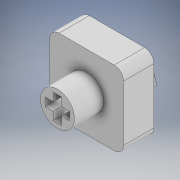
# Autodesk Inventor part: IPC ALOW 2 key
Saved by Autodesk Inventor 2022 (Build 260153000, 153)
## iProperties
Created: 2021-12-31
Part Number: IPC ALOW 2 key
Material: Generic
Document SubType Name: Modeling
Designer: solor
Density: 1 g/cm^3
Appearance: Default
Author: solor
Autodesk Inventor part; units mm, degrees
ref_plane "YZ Plane" through (0, 0, 0) normal (1, 0, 0) x (0, 1, 0)
ref_plane "XZ Plane" through (0, 0, 0) normal (0, 1, 0) x (-1, 0, 0)
sketch "Sketch1" plane through (0, 0, 0) normal (0, 0, 1) x (1, 0, 0)
  line L0 (14.6962, 12.74) -> (14.6962, 0) construction
  line L1 (10.61, 12.2) -> (1.53, 12.2)
  arc A0 (1.53, 12.2) -> (0, 10.67) centre (1.53, 10.67) ccw
  line L2 (0, 10.67) -> (0, 1.53)
  arc A1 (0, 1.53) -> (1.53, 0) centre (1.53, 1.53) ccw
  line L3 (1.53, 0) -> (10.61, 0)
  arc A2 (10.61, 0) -> (12.14, 1.53) centre (10.61, 1.53) ccw
  arc A3 (12.14, 10.67) -> (10.61, 12.2) centre (10.61, 10.67) ccw
  line L4 (12.14, 10.67) -> (12.14, 1.53)
  point P0 (0, 0)
  point P1 (0, 0)
  dimension "d10" = 12.74
  constraints: 10 end point, 8 point on circle, 4 centre point, 2 vertical, 1 point on line
  measures "d10" distance of L0.start L0.end
ref_plane "Work Plane1" through (0, 0, 5) normal (0, 0, 1) x (1, 0, 0)
sketch "Sketch2" plane through (0, 0, 5) normal (0, 0, 1) x (1, 0, 0)
  line L0 (10.88, 12.74) -> (1.8, 12.74) projected
  line L1 (10.88, 12.74) -> (1.8, 12.74) projected
  arc A0 (1.8, 12.74) -> (0, 10.94) centre (1.8, 10.94) ccw projected
  line L2 (0, 10.94) -> (0, 1.8) projected
  arc A1 (0, 1.8) -> (1.8, 0) centre (1.8, 1.8) ccw projected
  line L3 (1.8, 0) -> (10.88, 0) projected
  arc A2 (10.88, 0) -> (12.68, 1.8) centre (10.88, 1.8) ccw projected
  line L4 (12.68, 1.8) -> (12.68, 10.94) projected
  arc A3 (12.68, 10.94) -> (10.88, 12.74) centre (10.88, 10.94) ccw projected
  circle A4 centre (6.34, 6.37) radius 2.8
  line L5 (5.665, 8.395) -> (7.015, 8.395)
  line L6 (7.015, 4.345) -> (5.665, 4.345)
  line L7 (5.665, 4.345) -> (7.015, 8.395) construction
  line L8 (5.665, 8.395) -> (7.015, 4.345) construction
  line L9 (8.365, 5.695) -> (8.365, 7.045)
  line L10 (4.315, 7.045) -> (4.315, 5.695)
  line L11 (4.315, 5.695) -> (8.365, 7.045) construction
  line L12 (8.365, 5.695) -> (4.315, 7.045) construction
  line L13 (4.315, 5.695) -> (5.665, 5.695)
  line L14 (7.015, 5.695) -> (8.365, 5.695)
  line L15 (5.665, 4.345) -> (5.665, 5.695)
  line L16 (5.665, 7.045) -> (5.665, 8.395)
  line L17 (8.365, 7.045) -> (7.015, 7.045)
  line L18 (5.665, 7.045) -> (4.315, 7.045)
  line L19 (7.015, 8.395) -> (7.015, 7.045)
  line L20 (7.015, 5.695) -> (7.015, 4.345)
  point P0 (0, 0)
  dimension "d3" = 5.6
  dimension "d4" = 4.05
  dimension "d5" = 1.35
  dimension "d6" = 4.05
  dimension "d7" = 1.35
  constraints: 32 end point, 10 parallel, 8 perpendicular, 4 midpoint, 2 vertical, 1 centre point
  measures "d3" diameter of A4
  measures "d4" distance of L6.end L5.start
  measures "d5" distance of L5.start L5.end
  measures "d6" distance of L10.end L9.start
  measures "d7" distance of L9.end L9.start
extrude "Extrusion3" add sketch "Sketch1" along normal blind 5
sketch "Sketch3" plane through (0, 0, 5) normal (0, 0, 1) x (1, 0, 0)
  line L0 (10.61, 12.47) -> (1.53, 12.47)
  line L1 (10.61, 12.47) -> (1.53, 12.47)
  arc A0 (1.53, 12.47) -> (-0.27, 10.67) centre (1.53, 10.67) ccw
  line L2 (-0.27, 10.67) -> (-0.27, 1.53)
  arc A1 (-0.27, 1.53) -> (1.53, -0.27) centre (1.53, 1.53) ccw
  line L3 (1.53, -0.27) -> (10.61, -0.27)
  arc A2 (10.61, -0.27) -> (12.41, 1.53) centre (10.61, 1.53) ccw
  line L4 (12.41, 1.53) -> (12.41, 10.67)
  arc A3 (12.41, 10.67) -> (10.61, 12.47) centre (10.61, 10.67) ccw
  circle A4 centre (6.07, 6.1) radius 2.8
  line L5 (5.395, 8.125) -> (6.745, 8.125)
  line L6 (6.745, 4.075) -> (5.395, 4.075)
  line L7 (5.395, 4.075) -> (6.745, 8.125) construction
  line L8 (5.395, 8.125) -> (6.745, 4.075) construction
  line L9 (8.095, 5.425) -> (8.095, 6.775)
  line L10 (4.045, 6.775) -> (4.045, 5.425)
  line L11 (4.045, 5.425) -> (8.095, 6.775) construction
  line L12 (8.095, 5.425) -> (4.045, 6.775) construction
  line L13 (4.045, 5.425) -> (5.395, 5.425)
  line L14 (6.745, 5.425) -> (8.095, 5.425)
  line L15 (5.395, 4.075) -> (5.395, 5.425)
  line L16 (5.395, 6.775) -> (5.395, 8.125)
  line L17 (8.095, 6.775) -> (6.745, 6.775)
  line L18 (5.395, 6.775) -> (4.045, 6.775)
  line L19 (6.745, 8.125) -> (6.745, 6.775)
  line L20 (6.745, 5.425) -> (6.745, 4.075)
  line L21 (10.61, 12.2) -> (1.53, 12.2) projected
  line L22 (0, 10.67) -> (0, 1.53) projected
  point P0 (0, 0)
  point P1 (-0.27, -0.27)
  point P2 (6.07, 12.2)
  point P3 (0, 6.1)
  point P4 (6.07, 6.1)
  dimension "d14" = 5.6
  dimension "d15" = 4.05
  dimension "d16" = 1.35
  dimension "d17" = 4.05
  dimension "d18" = 1.35
  constraints: 42 end point, 10 parallel, 8 perpendicular, 8 point on circle, 6 midpoint, 5 centre point, 2 vertical
  measures "d14" diameter of A4
  measures "d15" distance of L6.end L5.start
  measures "d16" distance of L5.start L5.end
  measures "d17" distance of L10.end L9.start
  measures "d18" distance of L9.end L9.start
extrude "Extrusion4" add sketch "Sketch3" along normal blind 4.8 contours A4
sketch "Sketch4" plane through (0, 0, 0) normal (0, 0, -1) x (-1, 0, 0)
  line L0 (-1.53, 0) -> (-10.61, 0) projected
  line L1 (-11.7223, 9.7129) -> (-0.4177, 9.7129) construction
  line L2 (-0.4177, 9.7129) -> (-0.4177, 6.84) construction
  line L3 (-0.4177, 6.84) -> (-11.7223, 6.84) construction
  line L4 (-11.7223, 6.84) -> (-11.7223, 9.7129) construction
  line L5 (-7.4059, 5.3753) -> (-4.7341, 5.3753) construction
  line L6 (-4.7341, 5.3753) -> (-4.7341, 2.266) construction
  line L7 (-4.7341, 2.266) -> (-7.4059, 2.266) construction
  line L8 (-7.4059, 2.266) -> (-7.4059, 5.3753) construction
  line L9 (-11.7333, 6.956) -> (-10.8209, 9.656)
  line L10 (-10.8209, 9.656) -> (-10.0813, 9.656)
  line L11 (-10.0813, 9.656) -> (-9.1689, 6.956)
  line L12 (-9.1689, 6.956) -> (-9.8669, 6.956)
  line L13 (-9.8669, 6.956) -> (-10.0354, 7.5074)
  line L14 (-10.0354, 7.5074) -> (-10.8843, 7.5074)
  line L15 (-10.8843, 7.5074) -> (-11.055, 6.956)
  line L16 (-11.055, 6.956) -> (-11.7333, 6.956)
  line L17 (-10.1842, 7.9975) -> (-10.4598, 8.8902)
  line L18 (-10.4598, 8.8902) -> (-10.7377, 7.9975)
  line L19 (-10.7377, 7.9975) -> (-10.1842, 7.9975)
  line L20 (-7.0991, 6.956) -> (-8.8998, 6.956)
  line L21 (-8.8998, 6.956) -> (-8.8998, 9.656)
  line L22 (-8.8998, 9.656) -> (-8.2215, 9.656)
  line L23 (-8.2215, 9.656) -> (-8.2215, 7.4702)
  line L24 (-8.2215, 7.4702) -> (-7.0991, 7.4702)
  line L25 (-7.0991, 7.4702) -> (-7.0991, 6.956)
  spline S0 degree 2 poles (-4.3181, 8.306) (-4.3181, 7.6496) (-5.0183, 6.8991) (-5.6265, 6.8991) knots 0 0 0 1 2 2 2
  spline S1 degree 2 poles (-5.6265, 6.8991) (-6.237, 6.8991) (-6.9328, 7.6584) (-6.9328, 8.306) knots 0 0 0 1 2 2 2
  spline S2 degree 2 poles (-6.9328, 8.306) (-6.9328, 8.9559) (-6.237, 9.7129) (-5.6265, 9.7129) knots 0 0 0 1 2 2 2
  spline S3 degree 2 poles (-5.6265, 9.7129) (-5.0183, 9.7129) (-4.3181, 8.9602) (-4.3181, 8.306) knots 0 0 0 1 2 2 2
  spline S4 degree 2 poles (-5.0183, 8.306) (-5.0183, 8.5489) (-5.1167, 8.888) (-5.2021, 8.9952) knots 0 0 0 1 2 2 2
  spline S5 degree 2 poles (-5.2021, 8.9952) (-5.2874, 9.1068) (-5.5062, 9.2031) (-5.6243, 9.2031) knots 0 0 0 1 2 2 2
  spline S6 degree 2 poles (-5.6243, 9.2031) (-5.7491, 9.2031) (-5.9525, 9.1134) (-6.0466, 8.9996) knots 0 0 0 1 2 2 2
  spline S7 degree 2 poles (-6.0466, 8.9996) (-6.1298, 8.8946) (-6.2326, 8.5467) (-6.2326, 8.306) knots 0 0 0 1 2 2 2
  spline S8 degree 2 poles (-6.2326, 8.306) (-6.2326, 8.0566) (-6.1342, 7.7284) (-6.0488, 7.6168) knots 0 0 0 1 2 2 2
  spline S9 degree 2 poles (-6.0488, 7.6168) (-5.9635, 7.5052) (-5.7425, 7.4089) (-5.6243, 7.4089) knots 0 0 0 1 2 2 2
  spline S10 degree 2 poles (-5.6243, 7.4089) (-5.504, 7.4089) (-5.2808, 7.5118) (-5.1999, 7.6212) knots 0 0 0 1 2 2 2
  spline S11 degree 2 poles (-5.1999, 7.6212) (-5.1124, 7.7393) (-5.0183, 8.0522) (-5.0183, 8.306) knots 0 0 0 1 2 2 2
  line L26 (-0.4344, 9.656) -> (-1.1171, 6.956)
  line L27 (-1.1171, 6.956) -> (-1.861, 6.956)
  line L28 (-1.861, 6.956) -> (-2.2942, 8.6255)
  line L29 (-2.2942, 8.6255) -> (-2.7121, 6.956)
  line L30 (-2.7121, 6.956) -> (-3.4582, 6.956)
  line L31 (-3.4582, 6.956) -> (-4.1409, 9.656)
  line L32 (-4.1409, 9.656) -> (-3.4363, 9.656)
  line L33 (-3.4363, 9.656) -> (-3.0644, 7.8487)
  line L34 (-3.0644, 7.8487) -> (-2.6136, 9.656)
  line L35 (-2.6136, 9.656) -> (-1.9397, 9.656)
  line L36 (-1.9397, 9.656) -> (-1.5109, 7.8465)
  line L37 (-1.5109, 7.8465) -> (-1.1214, 9.656)
  line L38 (-1.1214, 9.656) -> (-0.4344, 9.656)
  line L39 (-4.8552, 2.266) -> (-7.097, 2.266)
  line L40 (-7.097, 2.266) -> (-7.097, 2.7628)
  spline S12 degree 2 poles (-7.097, 2.7628) (-6.8127, 2.9902) (-6.3579, 3.3906) (-6.1874, 3.571) knots 0 0 0 1 2 2 2
  spline S13 degree 2 poles (-6.1874, 3.571) (-5.9625, 3.8058) (-5.7623, 4.1642) (-5.7623, 4.3521) knots 0 0 0 1 2 2 2
  spline S14 degree 2 poles (-5.7623, 4.3521) (-5.7623, 4.5646) (-6.0169, 4.792) (-6.2443, 4.792) knots 0 0 0 1 2 2 2
  spline S15 degree 2 poles (-6.2443, 4.792) (-6.3604, 4.792) (-6.568, 4.7352) (-6.6743, 4.6907) knots 0 0 0 1 2 2 2
  spline S16 degree 2 poles (-6.6743, 4.6907) (-6.7781, 4.6437) (-6.9264, 4.5448) (-6.9635, 4.5201) knots 0 0 0 1 2 2 2
  line L41 (-6.9635, 4.5201) -> (-7.0228, 4.5201)
  line L42 (-7.0228, 4.5201) -> (-7.0228, 5.185)
  spline S17 degree 2 poles (-7.0228, 5.185) (-6.8943, 5.2468) (-6.3456, 5.3753) (-6.091, 5.3753) knots 0 0 0 1 2 2 2
  spline S18 degree 2 poles (-6.091, 5.3753) (-5.5472, 5.3753) (-4.9887, 4.8909) (-4.9887, 4.4534) knots 0 0 0 1 2 2 2
  spline S19 degree 2 poles (-4.9887, 4.4534) (-4.9887, 4.184) (-5.2432, 3.6649) (-5.5374, 3.3684) knots 0 0 0 1 2 2 2
  spline S20 degree 2 poles (-5.5374, 3.3684) (-5.7227, 3.1854) (-6.0712, 2.9012) (-6.1479, 2.8419) knots 0 0 0 1 2 2 2
  line L43 (-6.1479, 2.8419) -> (-4.8552, 2.8419)
  line L44 (-4.8552, 2.8419) -> (-4.8552, 2.266)
  point P0 (0, 0)
  point P1 (-6.07, 2.266)
  point P2 (-6.07, 6.84)
  point P3 (-6.07, 6.84)
  point P4 (-6.07, 2.266)
  constraints: 2 midpoint, 4 other
extrude "Extrusion5" add sketch "Sketch4" along normal blind 0.9
body "Solid2"
